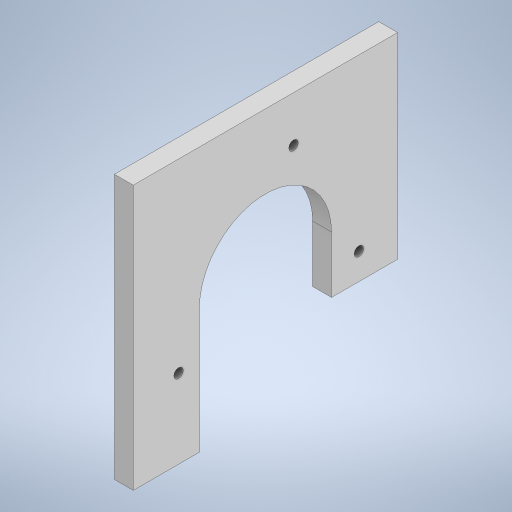
# Autodesk Inventor part: Двигатель ущербный
Saved by Autodesk Inventor 2023 (Build 270158000, 158)
## iProperties
Created: 2022-05-13
Part Number: Двигатель ущербный
Material: Типовые
Document SubType Name: Modeling
Designer: avkap
Density: 1 g/cm^3
Appearance: По умолчанию
Author: avkap
Autodesk Inventor part; units mm, degrees
ref_plane "YZ Plane" through (0, 0, 0) normal (1, 0, 0) x (0, 1, 0)
ref_plane "РабПлоскость8" through (-15, 0, 0) normal (-1, 0, 0) x (0, 0, 1)
sketch "Эскиз6" plane through (-15, 0, 0) normal (-1, 0, 0) x (0, 0, 1)
  line L0 (0, 0) -> (0, -66)
  line L1 (0, -66) -> (-70, -66)
  line L2 (-70, -66) -> (-70, 74)
  line L3 (-70, 74) -> (70, 74)
  line L4 (70, 74) -> (70, -66)
  line L5 (70, -66) -> (0, -66)
  circle A0 centre (0, 0) radius 3 projected
  circle A1 centre (-14.8513, 49.8341) radius 2.5 projected
  circle A2 centre (0, 0) radius 52
  line L6 (70, 0) -> (70, 30)
  line L7 (70, 0) -> (70, -20)
  circle A3 centre (0, 0) radius 35
  circle A4 centre (0, 0) radius 35 projected
  line L8 (0, 0) -> (70, 0)
  circle A5 centre (-14.8513, 49.8341) radius 2.5
  line L9 (-70, 74) -> (-73, 74)
  line L10 (-70, 89) -> (-70, 74)
  line L11 (-70, 74) -> (-67, 74)
  line L12 (-67, 74) -> (-67, 89)
  line L13 (-67, 89) -> (-70, 89)
  line L14 (-70, -66) -> (-70, -81)
  line L15 (-70, -81) -> (-67, -81)
  line L16 (-67, -81) -> (-67, -66)
  circle A6 centre (46.0282, -24.1951) radius 2.5 projected
  circle A7 centre (46.0282, -24.1951) radius 2.5
  line L17 (0, 74) -> (-30, 74)
  line L18 (-35, 0) -> (-35, 74)
  line L19 (-35, 0) -> (-35, -30)
  line L20 (-35, -30) -> (-70, -30)
  line L21 (35, 0) -> (35, -66)
  arc A8 (-56.6592, -9.0725) -> (-41.4997, -22.0629) centre (-49.4698, -16.0232) ccw projected
  circle A9 centre (-49.4698, -16.0232) radius 2.5
  point P0 (-1.4375, -51.9801)
  point P1 (38.1911, 35.2908)
  point P2 (0, -35)
  point P3 (35, 0)
  dimension "d36" = 66
  dimension "d37" = 70
  dimension "d38" = 140
  dimension "d39" = 140
  dimension "d45" = 3
  dimension "d46" = 15
  dimension "d47" = 15
  dimension "d48" = 3
  dimension "d49" = 30
  dimension "d54" = 30
  constraints: 44 end point, 12 point on line, 10 perpendicular, 5 coincident, 4 centre point, 3 midpoint, 2 horizontal, 2 vertical, 1 horizontal alignment, 1 tangent, 4 other
  measures "d36" distance of L0.start L0.end
  measures "d37" distance of L0.end L1.end
  measures "d38" distance of L1.end L2.end
  measures "d39" distance of L2.end L3.end
  measures "d45" distance of L2.end L11.end
  measures "d46" distance of L11.end L12.end
  measures "d47" distance of L1.end L14.end
  measures "d48" distance of L14.end L15.end
  measures "d49" distance of L17.start L17.end
  measures "d54" distance of L18.start L19.end
extrude "Выдавливание5" add sketch "Эскиз6" along normal blind 10 contours A3 L18 A2 A1 L8 | L8 A2 A6 L21 | L19 L20 A2 A9 L18 | L8 L4 L5 L21 A2 A6 | A2 A1 L18 L3 L4 L8 | L20 L2 L3 L18 A2 A9
ref_plane "РабПлоскость7" through (-25, 0, 0) normal (-1, 0, 0) x (0, 0, 1)
sketch "Эскиз7" plane through (-25, 0, 0) normal (-1, 0, 0) x (0, 0, 1)
  line L0 (-70, 74) -> (-70, -30) projected
  line L1 (-70, -30) -> (-35, -30) projected
  line L2 (-35, -30) -> (-35, 0) projected
  circle A0 centre (-49.4698, -16.0232) radius 2.5 projected
  arc A1 (35, 0) -> (-35, 0) centre (0, 0) ccw projected
  line L3 (70, 74) -> (-70, 74) projected
  line L4 (70, -66) -> (70, 74) projected
  line L5 (35, 0) -> (35, -66) projected
  line L6 (35, -66) -> (70, -66) projected
  circle A2 centre (46.0282, -24.1951) radius 2.5 projected
  circle A3 centre (-14.8513, 49.8341) radius 2.5 projected
  circle A4 centre (0, 0) radius 3 projected
  circle A5 centre (-14.8513, 49.8341) radius 2.5 projected
  circle A6 centre (0, 0) radius 52
  circle A7 centre (0, 0) radius 43.5 projected
  circle A8 centre (0, 0) radius 43.5 projected
  circle A9 centre (46.0282, -24.1951) radius 2.5 projected
  line L7 (0, 0) -> (46.0282, -24.1951)
  line L8 (46.0282, -24.1951) -> (46.0282, 0)
  line L9 (-14.8513, 49.8341) -> (0, 49.8341)
  arc A10 (28.4229, 37.4318) -> (-5.3572, 46.6937) centre (0, 0) ccw projected
  line L10 (0, 49.8341) -> (0, 0)
  circle A11 centre (-49.4698, -16.0232) radius 2.5 projected
  line L11 (0, 0) -> (-49.4698, -16.0232)
  line L12 (-49.4698, -16.0232) -> (-49.4995, -0.2197)
  circle A12 centre (-51.9995, -0.2244) radius 2.5 projected
  dimension "d57" = 104
  dimension "d55" = 104
  dimension "d56" = 140
  dimension "d58" = 35
  dimension "d59" = 87
  dimension "d60" = 24.1951
  dimension "d61" = 46.0282
  dimension "d62" = 49.8341
  dimension "d63" = 14.8513
  dimension "d64" = 15.8034
  dimension "d65" = 49.4999
  constraints: 12 end point, 1 coincident, 1 horizontal, 1 perpendicular, 1 vertical, 6 other
  measures "d55" distance of L0.start L0.end
  measures "d56" distance of L3.start L0.start
  measures "d58" radius of A1
  measures "d59" diameter of A8
  measures "d60" distance of L7.end L8.end
  measures "d61" distance of L8.end A1.centre
  measures "d62" distance of L9.end L10.end
  measures "d63" distance of L9.start L9.end
  measures "d64" distance of L11.end L12.end
  measures "d65" distance from line of L12 point (0, 0)
